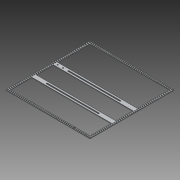
# Autodesk Inventor part: Rebuild Shooter Main Base
Saved by Autodesk Inventor 2014 SP1 (Build 180222100, 222)
## iProperties
Created: 2013-10-27
Part Number: Rebuild Shooter Main Base
Material: Aluminum 6061
Document SubType Name: Modeling
Designer: Moses
Density: 2.71 g/cm^3
Appearance: Aluminum - Flat
Mass: 322.056 g
Surface Area: 1094.46 cm^2
Volume: 118.84 cm^3
Author: Moses
Autodesk Inventor part; units mm, degrees
ref_plane "YZ Plane" through (0, 0, 0) normal (1, 0, 0) x (0, 1, 0)
ref_plane "XZ Plane" through (0, 0, 0) normal (0, 1, 0) x (-1, 0, 0)
ref_plane "XY Plane" through (0, 0, 0) normal (0, 0, 1) x (1, 0, 0)
sketch "Sketch1" plane through (0, 0, 0) normal (0, 1, 0) x (-1, 0, 0)
  line L0 (0, 0) -> (495.3, 0)
  line L1 (495.3, 0) -> (495.3, -495.3)
  line L2 (495.3, -495.3) -> (0, -495.3)
  line L3 (0, -495.3) -> (0, 0)
  line L4 (482.6, -12.7) -> (12.7, -12.7)
  line L5 (12.7, -12.7) -> (12.7, -482.6)
  line L6 (12.7, -482.6) -> (482.6, -482.6)
  line L7 (482.6, -482.6) -> (482.6, -12.7)
  circle A0 centre (6.35, -6.35) radius 3.3782
  circle A1 centre (16.199, -6.35) radius 3.3782
  circle A2 centre (26.048, -6.35) radius 3.3782
  circle A3 centre (35.8969, -6.35) radius 3.3782
  circle A4 centre (45.7459, -6.35) radius 3.3782
  circle A5 centre (55.5949, -6.35) radius 3.3782
  circle A6 centre (65.4439, -6.35) radius 3.3782
  circle A7 centre (75.2929, -6.35) radius 3.3782
  circle A8 centre (85.1418, -6.35) radius 3.3782
  circle A9 centre (94.9908, -6.35) radius 3.3782
  circle A10 centre (104.8398, -6.35) radius 3.3782
  circle A11 centre (114.6888, -6.35) radius 3.3782
  circle A12 centre (124.5378, -6.35) radius 3.3782
  circle A13 centre (134.3867, -6.35) radius 3.3782
  circle A14 centre (144.2357, -6.35) radius 3.3782
  circle A15 centre (154.0847, -6.35) radius 3.3782
  circle A16 centre (163.9337, -6.35) radius 3.3782
  circle A17 centre (173.7827, -6.35) radius 3.3782
  circle A18 centre (183.6316, -6.35) radius 3.3782
  circle A19 centre (193.4806, -6.35) radius 3.3782
  circle A20 centre (203.3296, -6.35) radius 3.3782
  circle A21 centre (213.1786, -6.35) radius 3.3782
  circle A22 centre (223.0276, -6.35) radius 3.3782
  circle A23 centre (232.8765, -6.35) radius 3.3782
  circle A24 centre (242.7255, -6.35) radius 3.3782
  circle A25 centre (252.5745, -6.35) radius 3.3782
  circle A26 centre (262.4235, -6.35) radius 3.3782
  circle A27 centre (272.2724, -6.35) radius 3.3782
  circle A28 centre (282.1214, -6.35) radius 3.3782
  circle A29 centre (291.9704, -6.35) radius 3.3782
  circle A30 centre (301.8194, -6.35) radius 3.3782
  circle A31 centre (311.6684, -6.35) radius 3.3782
  circle A32 centre (321.5173, -6.35) radius 3.3782
  circle A33 centre (331.3663, -6.35) radius 3.3782
  circle A34 centre (341.2153, -6.35) radius 3.3782
  circle A35 centre (351.0643, -6.35) radius 3.3782
  circle A36 centre (360.9133, -6.35) radius 3.3782
  circle A37 centre (370.7622, -6.35) radius 3.3782
  circle A38 centre (380.6112, -6.35) radius 3.3782
  circle A39 centre (390.4602, -6.35) radius 3.3782
  circle A40 centre (400.3092, -6.35) radius 3.3782
  circle A41 centre (410.1582, -6.35) radius 3.3782
  circle A42 centre (420.0071, -6.35) radius 3.3782
  circle A43 centre (429.8561, -6.35) radius 3.3782
  circle A44 centre (439.7051, -6.35) radius 3.3782
  circle A45 centre (449.5541, -6.35) radius 3.3782
  circle A46 centre (459.4031, -6.35) radius 3.3782
  circle A47 centre (469.252, -6.35) radius 3.3782
  circle A48 centre (479.101, -6.35) radius 3.3782
  circle A49 centre (488.95, -6.35) radius 3.3782
  circle A50 centre (6.35, -488.95) radius 3.3782
  circle A51 centre (16.199, -488.95) radius 3.3782
  circle A52 centre (26.048, -488.95) radius 3.3782
  circle A53 centre (35.8969, -488.95) radius 3.3782
  circle A54 centre (45.7459, -488.95) radius 3.3782
  circle A55 centre (55.5949, -488.95) radius 3.3782
  circle A56 centre (65.4439, -488.95) radius 3.3782
  circle A57 centre (75.2929, -488.95) radius 3.3782
  circle A58 centre (85.1418, -488.95) radius 3.3782
  circle A59 centre (94.9908, -488.95) radius 3.3782
  circle A60 centre (104.8398, -488.95) radius 3.3782
  circle A61 centre (114.6888, -488.95) radius 3.3782
  circle A62 centre (124.5378, -488.95) radius 3.3782
  circle A63 centre (134.3867, -488.95) radius 3.3782
  circle A64 centre (144.2357, -488.95) radius 3.3782
  circle A65 centre (154.0847, -488.95) radius 3.3782
  circle A66 centre (163.9337, -488.95) radius 3.3782
  circle A67 centre (173.7827, -488.95) radius 3.3782
  circle A68 centre (183.6316, -488.95) radius 3.3782
  circle A69 centre (193.4806, -488.95) radius 3.3782
  circle A70 centre (203.3296, -488.95) radius 3.3782
  circle A71 centre (213.1786, -488.95) radius 3.3782
  circle A72 centre (223.0276, -488.95) radius 3.3782
  circle A73 centre (232.8765, -488.95) radius 3.3782
  circle A74 centre (242.7255, -488.95) radius 3.3782
  circle A75 centre (252.5745, -488.95) radius 3.3782
  circle A76 centre (262.4235, -488.95) radius 3.3782
  circle A77 centre (272.2724, -488.95) radius 3.3782
  circle A78 centre (282.1214, -488.95) radius 3.3782
  circle A79 centre (291.9704, -488.95) radius 3.3782
  circle A80 centre (301.8194, -488.95) radius 3.3782
  circle A81 centre (311.6684, -488.95) radius 3.3782
  circle A82 centre (321.5173, -488.95) radius 3.3782
  circle A83 centre (331.3663, -488.95) radius 3.3782
  circle A84 centre (341.2153, -488.95) radius 3.3782
  circle A85 centre (351.0643, -488.95) radius 3.3782
  circle A86 centre (360.9133, -488.95) radius 3.3782
  circle A87 centre (370.7622, -488.95) radius 3.3782
  circle A88 centre (380.6112, -488.95) radius 3.3782
  circle A89 centre (390.4602, -488.95) radius 3.3782
  circle A90 centre (400.3092, -488.95) radius 3.3782
  circle A91 centre (410.1582, -488.95) radius 3.3782
  circle A92 centre (420.0071, -488.95) radius 3.3782
  circle A93 centre (429.8561, -488.95) radius 3.3782
  circle A94 centre (439.7051, -488.95) radius 3.3782
  circle A95 centre (449.5541, -488.95) radius 3.3782
  circle A96 centre (459.4031, -488.95) radius 3.3782
  circle A97 centre (469.252, -488.95) radius 3.3782
  circle A98 centre (479.101, -488.95) radius 3.3782
  circle A99 centre (488.95, -488.95) radius 3.3782
  circle A100 centre (6.35, -17.4171) radius 3.3782
  circle A101 centre (488.95, -17.4171) radius 3.3782
  circle A102 centre (6.35, -28.4843) radius 3.3782
  circle A103 centre (488.95, -28.4843) radius 3.3782
  circle A104 centre (6.35, -39.5514) radius 3.3782
  circle A105 centre (488.95, -39.5514) radius 3.3782
  circle A106 centre (6.35, -50.6186) radius 3.3782
  circle A107 centre (488.95, -50.6186) radius 3.3782
  circle A108 centre (6.35, -61.6857) radius 3.3782
  circle A109 centre (488.95, -61.6857) radius 3.3782
  circle A110 centre (6.35, -72.7529) radius 3.3782
  circle A111 centre (488.95, -72.7529) radius 3.3782
  circle A112 centre (6.35, -83.82) radius 3.3782
  circle A113 centre (488.95, -83.82) radius 3.3782
  circle A114 centre (6.35, -94.8871) radius 3.3782
  circle A115 centre (488.95, -94.8871) radius 3.3782
  circle A116 centre (6.35, -105.9543) radius 3.3782
  circle A117 centre (488.95, -105.9543) radius 3.3782
  circle A118 centre (6.35, -117.0214) radius 3.3782
  circle A119 centre (488.95, -117.0214) radius 3.3782
  circle A120 centre (6.35, -128.0886) radius 3.3782
  circle A121 centre (488.95, -128.0886) radius 3.3782
  circle A122 centre (6.35, -139.1557) radius 3.3782
  circle A123 centre (488.95, -139.1557) radius 3.3782
  circle A124 centre (6.35, -150.2229) radius 3.3782
  circle A125 centre (488.95, -150.2229) radius 3.3782
  circle A126 centre (6.35, -161.29) radius 3.3782
  circle A127 centre (488.95, -161.29) radius 3.3782
  circle A128 centre (6.35, -172.3571) radius 3.3782
  circle A129 centre (488.95, -172.3571) radius 3.3782
  circle A130 centre (6.35, -183.4243) radius 3.3782
  circle A131 centre (488.95, -183.4243) radius 3.3782
  circle A132 centre (6.35, -194.4914) radius 3.3782
  circle A133 centre (488.95, -194.4914) radius 3.3782
  circle A134 centre (6.35, -205.5586) radius 3.3782
  circle A135 centre (488.95, -205.5586) radius 3.3782
  circle A136 centre (6.35, -216.6257) radius 3.3782
  circle A137 centre (488.95, -216.6257) radius 3.3782
  circle A138 centre (6.35, -227.6929) radius 3.3782
  circle A139 centre (488.95, -227.6929) radius 3.3782
  circle A140 centre (6.35, -238.76) radius 3.3782
  circle A141 centre (488.95, -238.76) radius 3.3782
  circle A142 centre (6.35, -249.8271) radius 3.3782
  circle A143 centre (488.95, -249.8271) radius 3.3782
  circle A144 centre (6.35, -260.8943) radius 3.3782
  circle A145 centre (488.95, -260.8943) radius 3.3782
  circle A146 centre (6.35, -271.9614) radius 3.3782
  circle A147 centre (488.95, -271.9614) radius 3.3782
  circle A148 centre (6.35, -283.0286) radius 3.3782
  circle A149 centre (488.95, -283.0286) radius 3.3782
  circle A150 centre (6.35, -294.0957) radius 3.3782
  circle A151 centre (488.95, -294.0957) radius 3.3782
  circle A152 centre (6.35, -305.1629) radius 3.3782
  circle A153 centre (488.95, -305.1629) radius 3.3782
  circle A154 centre (6.35, -316.23) radius 3.3782
  circle A155 centre (488.95, -316.23) radius 3.3782
  circle A156 centre (6.35, -327.2971) radius 3.3782
  circle A157 centre (488.95, -327.2971) radius 3.3782
  circle A158 centre (6.35, -338.3643) radius 3.3782
  circle A159 centre (488.95, -338.3643) radius 3.3782
  circle A160 centre (6.35, -349.4314) radius 3.3782
  circle A161 centre (488.95, -349.4314) radius 3.3782
  circle A162 centre (6.35, -360.4986) radius 3.3782
  circle A163 centre (488.95, -360.4986) radius 3.3782
  circle A164 centre (6.35, -371.5657) radius 3.3782
  circle A165 centre (488.95, -371.5657) radius 3.3782
  line L8 (12.7, -139.7) -> (482.6, -139.7)
  line L9 (482.6, -165.1) -> (12.7, -165.1)
  line L10 (12.7, -266.7) -> (482.6, -266.7)
  line L11 (482.6, -292.1) -> (12.7, -292.1)
  line L12 (247.65, -139.7) -> (247.65, -165.1) construction
  line L13 (247.65, -266.7) -> (247.65, -292.1) construction
  line L14 (12.7, -152.4) -> (482.6, -152.4) construction
  line L15 (12.7, -279.4) -> (482.6, -279.4) construction
  arc A166 (101.6, -149.0218) -> (101.6, -155.7782) centre (101.6, -152.4) ccw
  arc A167 (406.4, -155.7782) -> (406.4, -149.0218) centre (406.4, -152.4) ccw
  arc A168 (101.6, -276.0218) -> (101.6, -282.7782) centre (101.6, -279.4) ccw
  arc A169 (406.4, -282.7782) -> (406.4, -276.0218) centre (406.4, -279.4) ccw
  line L16 (101.6, -149.0218) -> (406.4, -149.0218)
  line L17 (406.4, -155.7782) -> (101.6, -155.7782)
  line L18 (101.6, -276.0218) -> (406.4, -276.0218)
  line L19 (406.4, -282.7782) -> (101.6, -282.7782)
  line L20 (12.7, -139.7) -> (12.7, -165.1)
  line L21 (12.7, -266.7) -> (12.7, -292.1)
  line L22 (482.6, -139.7) -> (482.6, -165.1)
  line L23 (482.6, -266.7) -> (482.6, -292.1)
  circle A170 centre (6.35, -382.6329) radius 3.3782
  circle A171 centre (488.95, -382.6329) radius 3.3782
  circle A172 centre (6.35, -477.0437) radius 3.3782
  circle A173 centre (488.95, -477.0437) radius 3.3782
  circle A174 centre (6.35, -465.1375) radius 3.3782
  circle A175 centre (488.95, -465.1375) radius 3.3782
  circle A176 centre (6.35, -453.2312) radius 3.3782
  circle A177 centre (488.95, -453.2312) radius 3.3782
  circle A178 centre (6.35, -441.325) radius 3.3782
  circle A179 centre (488.95, -441.325) radius 3.3782
  circle A180 centre (6.35, -429.4187) radius 3.3782
  circle A181 centre (488.95, -429.4187) radius 3.3782
  circle A182 centre (6.35, -417.5125) radius 3.3782
  circle A183 centre (488.95, -417.5125) radius 3.3782
  circle A184 centre (6.35, -405.6063) radius 3.3782
  circle A185 centre (488.95, -405.6063) radius 3.3782
  circle A186 centre (6.35, -393.7) radius 3.3782
  circle A187 centre (488.95, -393.7) radius 3.3782
  circle A188 centre (438.15, -279.4) radius 3.3782 projected
  circle A189 centre (469.9, -279.4) radius 3.3782 projected
  ellipse E0 centre (438.15, -152.3984) end of major axis (434.7718, -152.3984) minor radius 3.3782 projected
  ellipse E1 centre (469.9, -152.3984) end of major axis (473.2782, -152.3984) minor radius 3.3782 projected
  circle A190 centre (290.4658, -393.7) radius 3.3782 construction
  circle A191 centre (211.3506, -283.9494) radius 3.3782 construction
  circle A192 centre (235.1483, -260.1517) radius 3.3782 construction
  circle A193 centre (256.8108, -393.7) radius 3.3782 construction
  line L24 (230.7599, -246.5796) -> (370.8628, -106.4767) construction
  arc A194 (388.8233, -124.4372) -> (370.8628, -106.4767) centre (101.6, -393.7) ccw construction
  line L25 (388.8233, -124.4372) -> (135.9803, -377.2803) construction
  arc A195 (139.1671, -387.35) -> (135.9803, -377.2803) centre (101.6, -393.7) ccw construction
  line L26 (139.1671, -387.35) -> (495.2488, -387.35) construction
  arc A196 (495.3, -393.7) -> (495.2488, -387.35) centre (101.6, -393.7) ccw construction
  line L27 (495.3, -393.7) -> (495.3, -400.05) construction
  line L28 (495.3, -400.05) -> (139.1671, -400.05) construction
  arc A197 (95.25, -356.1329) -> (139.1671, -400.05) centre (101.6, -393.7) ccw construction
  line L29 (95.25, -356.1329) -> (95.25, -294.0283) construction
  arc A198 (95.25, -294.0283) -> (107.95, -279.2597) centre (-8.89, -191.6297) ccw construction
  line L30 (107.95, -279.2597) -> (173.6725, -191.6297) construction
  line L31 (173.6725, -191.6297) -> (107.95, -103.9997) construction
  arc A199 (107.95, -103.9997) -> (95.25, -89.2312) centre (-8.89, -191.6297) ccw construction
  line L32 (95.25, -89.2312) -> (95.25, 0) construction
  line L33 (95.25, 0) -> (101.6, 0) construction
  arc A200 (107.95, -0.0512) -> (101.6, 0) centre (101.6, -393.7) ccw construction
  line L34 (107.95, -0.0512) -> (107.95, -82.8331) construction
  line L35 (107.95, -82.8331) -> (230.7599, -246.5796) construction
  circle A201 centre (101.6, -6.35) radius 3.3782 construction
  circle A202 centre (101.6, -57.15) radius 3.3782 construction
  line L36 (221.6885, -255.651) -> (181.61, -202.2131) construction
  line L37 (181.61, -202.2131) -> (107.95, -300.4264) construction
  line L38 (107.95, -300.4264) -> (107.95, -356.1329) construction
  arc A203 (118.0197, -359.3197) -> (107.95, -356.1329) centre (101.6, -393.7) ccw construction
  line L39 (118.0197, -359.3197) -> (221.6885, -255.651) construction
  circle A204 centre (101.6, -393.7) radius 9.5 construction
  circle A205 centre (371.8276, -116.1805) radius 3.3782 construction
  circle A206 centre (379.1195, -123.4724) radius 3.3782 construction
  circle A207 centre (335.9065, -152.1015) radius 3.3782 construction
  circle A208 centre (343.1985, -159.3935) radius 3.3782 construction
  circle A209 centre (488.95, -393.7) radius 3.3782 construction
  circle A210 centre (438.15, -393.7) radius 3.3782 construction
  circle A211 centre (241.3, -393.7) radius 3.3782 construction
  circle A212 centre (381, -393.7) radius 3.3782 construction
  circle A213 centre (195.7906, -290.5292) radius 3.3782 construction
  circle A214 centre (204.7708, -299.5094) radius 3.3782 construction
  circle A215 centre (294.6245, -191.6953) radius 3.3782 construction
  circle A216 centre (303.6047, -200.6755) radius 3.3782 construction
  circle A217 centre (101.6, -6.35) radius 3.81
  point P0 (247.65, -152.4)
  point P1 (247.65, -279.4)
  dimension "d0" = 495.3
  dimension "d1" = 495.3
  dimension "d2" = 12.7
  dimension "d3" = 6.7564
  dimension "d4" = 6.35
  dimension "d5" = 6.35
  dimension "d8" = 9.849
  dimension "d11" = 482.6
  dimension "d16" = 11.0671
  dimension "d21" = 25.4
  dimension "d22" = 25.4
  dimension "d23" = 127
  dimension "d24" = 254
  dimension "d25" = 88.9
  dimension "d26" = 88.9
  dimension "d27" = 76.2
  dimension "d28" = 76.2
  dimension "d38" = 11.9062
  dimension "d43" = 11.0671
  dimension "d44" = 11.9062
  dimension "d45" = 7.62
  constraints: 189 centre point, 48 end point, 15 point on line, 8 midpoint, 8 perpendicular, 8 point on circle, 8 tangent, 5 parallel, 4 equal radius, 4 vertical, 3 collinear, 2 horizontal, 1 coincident, 371 other
  measures "d0" distance of L1.end L2.end
  measures "d1" distance of L0.end L1.end
  measures "d2" distance between parallel lines of L4 L0
  measures "d3" diameter of A0
  measures "d4" distance from line of L0 A0.centre
  measures "d5" distance from line of L3 A0.centre
  measures "d8" distance of A0.centre A1.centre
  measures "d11" distance of A0.centre A50.centre
  measures "d16" distance of A0.centre A100.centre
  measures "d21" distance of L11.end L10.start
  measures "d22" distance of L9.end L8.start
  measures "d23" distance of L4.start L8.end
  measures "d24" distance of L4.start L10.end
  measures "d25" distance of A166.centre L14.start
  measures "d26" distance of A168.centre L15.start
  measures "d27" distance of L14.end A167.centre
  measures "d28" distance of L15.end A169.centre
  measures "d38" distance of A50.centre A172.centre
  measures "d43" distance of A186.centre A170.centre
  measures "d44" distance of A186.centre A184.centre
  measures "d45" diameter of A217
extrude "Extrusion1" add sketch "Sketch1" along normal blind 3.175 contours L0 L1 L2 L3 | L7 L9 L5 L8 | L7 L11 L5 L10
equation "\"d8\" = -0.0408163 * d5 + 0.0204082 * d0"
equation "\"d11\" = d1 - 2 * d4"
equation "\"d21\" = d22"
equation "\"d26\" = d25"
body "Solid1"
